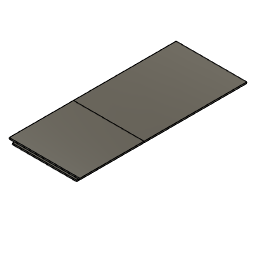
Modular RC Boat Hull (Autodesk Fusion 360 archive; units mm, degrees)
design "Modular RC Boat Top"
Autodesk Fusion 360 part; units mm, degrees
ref_plane "WorkPlane1" through (0, 0, 43) normal (0, 0, 1) x (1, 0, 0)
sketch "Sketch2" plane through (0, 0, 43) normal (0, 0, 1) x (1, 0, 0)
  line L0 (-50, 30) -> (50, 30)
  line L1 (50, 30) -> (50, -225)
  line L2 (50, -225) -> (-50, -225)
  line L3 (-50, -225) -> (-50, 30)
  constraint horizontal L0
  constraint vertical L1
  constraint horizontal L2
  constraint vertical L3
extrude "Extrude1" add sketch "Sketch2" along normal blind 2 makes body 1
sketch "Sketch3" plane through (0, 0, 45) normal (0, 0, 1) x (-1, 0, 0)
  line L0 (50, 225) -> (-50, 225)
  line L1 (-50, 225) -> (-50, -30)
  line L2 (-50, -30) -> (50, -30)
  line L3 (50, -30) -> (50, 225)
  line L4 (50, -30) -> (-50, -30)
  line L5 (-50, -30) -> (-50, 220)
  line L6 (-50, 220) -> (50, 220)
  line L7 (50, 220) -> (50, -30)
  constraint horizontal L4
  constraint vertical L5
  constraint horizontal L6
  constraint vertical L7
  constraint coincident L1 L5.end
  constraint coincident L2.end L3.start
extrude "Extrude2" add sketch "Sketch3" along normal blind 3 contours L1 L2 L3 L4 L5 L6 L7 bodies 1
sketch "Sketch4" plane through (0, 0, 48) normal (0, 0, 1) x (-1, 0, 0)
  line L0 (50, 220) -> (-50, 220)
  line L1 (-50, 220) -> (-50, -30)
  line L2 (-50, -30) -> (50, -30)
  line L3 (50, -30) -> (50, 220)
  line L4 (50, -30) -> (-50, -30)
  line L5 (-50, -30) -> (-50, 225)
  line L6 (-50, 225) -> (50, 225)
  line L7 (50, 225) -> (50, -30)
  line L8 (55, -35) -> (-55, -35)
  line L9 (-55, -35) -> (-55, 225)
  line L10 (-55, 225) -> (55, 225)
  line L11 (55, 225) -> (55, -35)
  constraint horizontal L4
  constraint vertical L5
  constraint horizontal L6
  constraint vertical L7
  constraint coincident L2.end L3.start
  constraint horizontal L8
  constraint vertical L9
  constraint horizontal L10
  constraint vertical L11
extrude "Extrude3" add sketch "Sketch4" along normal blind 2 bodies 1
ref_plane "WorkPlane3" through (0, -125, 0) normal (0, 1, 0) x (0, 0, 1)
split "Split1" by plane through (0, -125, 0) normal (0, 1, 0) bodies 1 makes body 2 at (18.3333, -71.6667, 50)
sketch "Sketch5" plane through (0, -125, 0) normal (0, -1, 0) x (1, 0, 0)
  line L0 (-55, 48) -> (-50, 48)
  line L1 (-50, 48) -> (-50, 43)
  line L2 (-50, 43) -> (50, 43)
  line L3 (50, 43) -> (50, 48)
  line L4 (50, 48) -> (55, 48)
  line L5 (55, 48) -> (55, 50)
  line L6 (55, 50) -> (-55, 50)
  line L7 (-55, 50) -> (-55, 48)
  line L8 (-45, 48) -> (45, 48)
  line L9 (45, 48) -> (45, 45)
  line L10 (45, 45) -> (-45, 45)
  line L11 (-45, 45) -> (-45, 48)
  constraint horizontal L8
  constraint vertical L9
  constraint horizontal L10
  constraint vertical L11
extrude "Extrude4" add sketch "Sketch5" along normal blind 19 contours L8 L9 L10 L11 bodies 2
sketch "Sketch6" plane through (0, -125, 0) normal (0, 1, 0) x (-1, 0, 0)
  line L0 (50, 48) -> (55, 48)
  line L1 (55, 48) -> (55, 50)
  line L2 (55, 50) -> (-55, 50)
  line L3 (-55, 50) -> (-55, 48)
  line L4 (-55, 48) -> (-50, 48)
  line L5 (-50, 48) -> (-50, 43)
  line L6 (-50, 43) -> (50, 43)
  line L7 (50, 43) -> (50, 48)
  line L8 (-45, 48) -> (45, 48)
  line L9 (45, 48) -> (45, 45)
  line L10 (45, 45) -> (-45, 45)
  line L11 (-45, 45) -> (-45, 48)
  constraint horizontal L8
  constraint vertical L9
  constraint horizontal L10
  constraint vertical L11
extrude "Extrude5" cut sketch "Sketch6" against normal blind 20 contours L8 L9 L10 L11 bodies 1
named bodies: "Top Segment 1", "Top Segment 2"

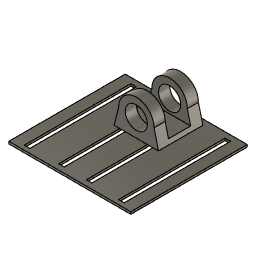
design "Modular RC Boat Motor Mount"
Autodesk Fusion 360 part; units mm, degrees
ref_plane "WorkPlane1" through (0, 0, 7) normal (0, 0, 1) x (1, 0, 0)
sketch "Sketch1" plane through (0, 0, 7) normal (0, 0, 1) x (1, 0, 0)
  line L0 (-15, -5) -> (-10, -5)
  line L1 (-10, -5) -> (-10, -100)
  line L2 (-10, -100) -> (-15, -100)
  line L3 (-15, -100) -> (-15, -5)
  line L4 (10, -100) -> (15, -100)
  line L5 (15, -100) -> (15, -5)
  line L6 (15, -5) -> (10, -5)
  line L7 (10, -5) -> (10, -100)
  line L8 (-55, 0) -> (55, 0)
  line L9 (55, 0) -> (55, -105)
  line L10 (55, -105) -> (-55, -105)
  line L11 (-55, -105) -> (-55, 0)
  line L12 (-40, -5) -> (-45, -5)
  line L13 (-45, -5) -> (-45, -101)
  line L14 (-45, -101) -> (-40, -101)
  line L15 (-40, -101) -> (-40, -5)
  line L16 (40, -5) -> (45, -5)
  line L17 (45, -5) -> (45, -101)
  line L18 (45, -101) -> (40, -101)
  line L19 (40, -101) -> (40, -5)
  constraint horizontal L0
  constraint vertical L1
  constraint horizontal L2
  constraint vertical L3
  constraint horizontal L4
  constraint vertical L5
  constraint horizontal L6
  constraint vertical L7
  constraint horizontal L8
  constraint vertical L9
  constraint horizontal L10
  constraint vertical L11
  constraint horizontal L12
  constraint vertical L13
  constraint horizontal L14
  constraint vertical L15
  constraint horizontal L16
  constraint vertical L17
  constraint horizontal L18
  constraint vertical L19
extrude "Extrude1" add sketch "Sketch1" along normal blind 2
ref_plane "WorkPlane2" through (0, -5, 0) normal (0, 1, 0) x (0, 0, 1)
sketch "Sketch2" plane through (0, -5, 0) normal (0, 1, 0) x (1, 0, 0)
  circle A0 centre (0, -25) radius 16
  circle A1 centre (0, -25) radius 10
  line L0 (-20, -9) -> (-16, -25)
  line L1 (-20, -9) -> (0, -9)
  line L2 (16, -25) -> (20, -9)
  line L3 (20, -9) -> (0, -9)
  dimension "d10" = 20
  constraint concentric A0 A1
  constraint coincident A0 L0.end
  constraint coincident A0 L1.end
  constraint tangent A0 L1
  constraint horizontal L1
  constraint coincident A0 L2.start
  constraint tangent A0 L3
  measures "d10" diameter of A1
extrude "Extrude2" add sketch "Sketch2" against normal blind 40
ref_plane "WorkPlane3" through (0, 0, 41) normal (0, 0, 1) x (1, 0, 0)
sketch "Sketch4" plane through (0, 0, 41) normal (0, 0, 1) x (1, 0, 0)
  line L0 (-20, -15) -> (20, -15)
  line L1 (20, -15) -> (20, -35)
  line L2 (20, -35) -> (-20, -35)
  line L3 (-20, -35) -> (-20, -15)
  constraint horizontal L0
  constraint vertical L1
  constraint horizontal L2
  constraint vertical L3
extrude "Extrude4" cut sketch "Sketch4" against normal blind 28
named bodies: "Mount"
